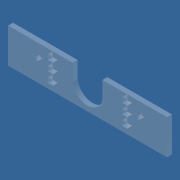
# Autodesk Inventor part: acrylic kinect bracket - kinect plate
Saved by Autodesk Inventor 2012 (Build 160160000, 160)
## iProperties
Created: 2012-11-01
Part Number: acrylic kinect bracket - kinect plate
Material: Default
Document SubType Name: Modeling
Designer: Ed
Density: 1 g/cm^3
Author: Ed
Autodesk Inventor part; units mm, degrees
ref_plane "YZ Plane" through (0, 0, 0) normal (1, 0, 0) x (0, 1, 0)
ref_plane "XZ Plane" through (0, 0, 0) normal (0, 1, 0) x (-1, 0, 0)
ref_plane "XY Plane" through (0, 0, 0) normal (0, 0, 1) x (1, 0, 0)
sketch "Sketch1" plane through (0, 0, 0) normal (0, 0, 1) x (1, 0, 0)
  line L0 (-101.6, -22.225) -> (101.6, -22.225)
  line L1 (101.6, -22.225) -> (101.6, 22.225)
  line L2 (101.6, 22.225) -> (-101.6, 22.225)
  line L3 (-101.6, 22.225) -> (-101.6, -22.225)
  line L4 (-19.05, 22.225) -> (-19.05, 3.175)
  arc A0 (-19.05, 3.175) -> (19.05, 3.175) centre (0, 3.175) ccw
  line L5 (19.05, 3.175) -> (19.05, 22.225)
  line L6 (-50.8, 15.875) -> (-44.45, 15.875)
  line L7 (-44.45, 15.875) -> (-44.45, 9.525)
  line L8 (-44.45, 9.525) -> (-50.8, 9.525)
  line L9 (-50.8, 9.525) -> (-50.8, 15.875)
  line L10 (44.45, 15.875) -> (50.8, 15.875)
  line L11 (50.8, 15.875) -> (50.8, 9.525)
  line L12 (50.8, 9.525) -> (44.45, 9.525)
  line L13 (44.45, 9.525) -> (44.45, 15.875)
  line L14 (-50.8, 3.175) -> (-44.45, 3.175)
  line L15 (-44.45, 3.175) -> (-44.45, -3.175)
  line L16 (-44.45, -3.175) -> (-50.8, -3.175)
  line L17 (-50.8, -3.175) -> (-50.8, 3.175)
  line L18 (44.45, 3.175) -> (50.8, 3.175)
  line L19 (50.8, 3.175) -> (50.8, -3.175)
  line L20 (50.8, -3.175) -> (44.45, -3.175)
  line L21 (44.45, -3.175) -> (44.45, 3.175)
  line L22 (-50.8, -9.525) -> (-44.45, -9.525)
  line L23 (-44.45, -9.525) -> (-44.45, -15.875)
  line L24 (-44.45, -15.875) -> (-50.8, -15.875)
  line L25 (-50.8, -15.875) -> (-50.8, -9.525)
  line L26 (44.45, -9.525) -> (50.8, -9.525)
  line L27 (50.8, -9.525) -> (50.8, -15.875)
  line L28 (50.8, -15.875) -> (44.45, -15.875)
  line L29 (44.45, -15.875) -> (44.45, -9.525)
  point P0 (0, 0)
  point P1 (-101.6, 0)
  point P2 (0, 22.225)
  dimension "d0" = 203.2
  dimension "d1" = 44.45
  dimension "d2" = 6.35
  dimension "d3" = 44.45
  dimension "d4" = 6.35
  dimension "d7" = 95.25
  dimension "d10" = 12.7
  dimension "d13" = 19.05
  dimension "d14" = 19.05
  constraints: 60 end point, 5 parallel, 4 perpendicular, 3 horizontal, 2 midpoint, 2 point on circle, 2 point on line, 2 tangent, 2 vertical alignment, 1 centre point, 1 horizontal alignment, 1 vertical, 40 other
  measures "d0" distance of L0.start L0.end
  measures "d1" distance of L2.end L0.start
  measures "d2" distance of L6.start L6.end
  measures "d3" distance from line of point (0, 22.225) L7
  measures "d4" distance between parallel lines of L2 L6
  measures "d7" distance of L6.start L10.start
  measures "d10" distance of L6.start L14.start
  measures "d13" radius of A0
  measures "d14" distance of L5.start L5.end
extrude "Extrusion1" add sketch "Sketch1" along normal blind 6.35 contours L3 L2 L4 A0 L5 L1 L0
sketch "Sketch2" plane through (0, 0, 6.35) normal (0, 0, 1) x (1, 0, 0)
  line L0 (101.6, -22.225) -> (-101.6, -22.225) projected
  point P0 (0, 0)
  point P1 (-65.0875, 3.175)
  point P2 (65.0875, 3.175)
  dimension "d18" = 65.0875
  dimension "d26" = 130.175
  dimension "d27" = 25.4
  constraints: 1 horizontal alignment
  measures "d18" horizontal distance of point (-65.088, 3.175) point (0, 0)
  measures "d26" distance of point (65.088, 3.175) point (-65.088, 3.175)
  measures "d27" distance from line of L0 point (-65.088, 3.175)
hole "Hole1" at (-65.0875, 3.175, 6.35) at (65.0875, 3.175, 6.35) direction (0, 0, -1) diameter 3.81 end through all clearance for "Flat Head Machine Screw (82)" size "#6" standard "Ansi Unified Screw Threads"
equation "\"d18\" = 0.5 * d26"
body "Solid1"
